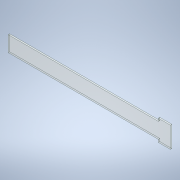
# Autodesk Inventor part: petg
Saved by Autodesk Inventor 2022 (Build 260153000, 153)
## iProperties
Created: 2024-02-25
Part Number: petg
Material: Genérico
Document SubType Name: Modeling
Designer: Daniel
Density: 1 g/cm^3
Appearance: Transparente
Author: Daniel
Autodesk Inventor part; units mm, degrees
ref_plane "YZ Plane" through (0, 0, 0) normal (1, 0, 0) x (0, 1, 0)
ref_plane "XZ Plane" through (0, 0, 0) normal (0, 1, 0) x (-1, 0, 0)
ref_plane "XY Plane" through (0, 0, 0) normal (0, 0, 1) x (1, 0, 0)
sketch "Esboço1" plane through (0, 0, 0) normal (0, 0, 1) x (1, 0, 0)
  line L0 (-2, -3.5) -> (2, -3.5)
  line L1 (2, -3.5) -> (2, 3.5)
  line L2 (2, 3.5) -> (-2, 3.5)
  line L3 (-2, 3.5) -> (-2, -3.5)
  line L4 (-2, -3.5) -> (2, 3.5) construction
  line L5 (2, -3.5) -> (-2, 3.5) construction
  line L6 (-2, -2.596) -> (-52, -2.596)
  line L7 (-52, -2.596) -> (-52, 0)
  line L8 (-7, 0) -> (14.596, 0)
  line L9 (-2, 2.596) -> (-52, 2.596)
  line L10 (-52, 2.596) -> (-52, 0)
  line L11 (0, 13.892) -> (0, -5.8963)
  point P0 (0, 0)
  point P1 (-2, 2.596)
  dimension "d3" = 4
  dimension "d4" = 7
  dimension "d5" = 50
  constraints: 24 end point, 3 horizontal, 2 parallel, 2 symmetric about line, 2 vertical, 1 perpendicular, 1 point on line
  measures "d3" distance of L2.end L1.end
  measures "d4" distance of L1.end L0.end
  measures "d5" distance of L6.start L6.end
extrude "Extrusão1" add sketch "Esboço1" along normal blind 0.5
